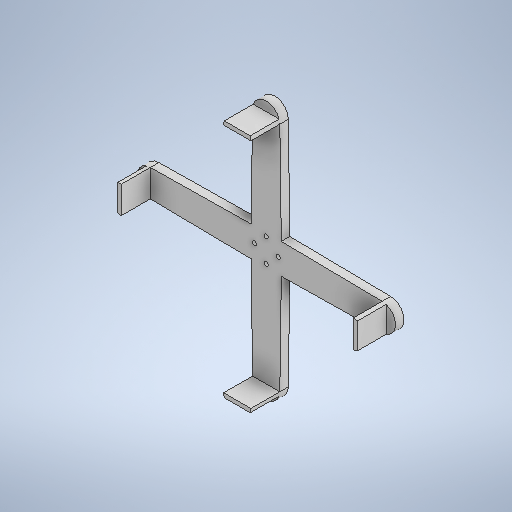
# Autodesk Inventor part: beadlock
Saved by Autodesk Inventor 2025.3 (Build 293356000, 356)
## iProperties
Created: 2026-03-16
Part Number: beadlock
Material: Generic
Document SubType Name: Modeling
Designer: ksawe
Density: 1 g/cm^3
Appearance: Default
Author: ksawe
Autodesk Inventor part; units mm, degrees
ref_plane "YZ Plane" through (0, 0, 0) normal (1, 0, 0) x (0, 1, 0)
ref_plane "XZ Plane" through (0, 0, 0) normal (0, 1, 0) x (-1, 0, 0)
ref_plane "XY Plane" through (0, 0, 0) normal (0, 0, 1) x (1, 0, 0)
sketch "Sketch1" plane through (0, 0, 0) normal (0, 0, 1) x (1, 0, 0)
  circle A0 centre (0, 0) radius 9 construction
  circle A1 centre (0, -7) radius 1.25
  circle A2 centre (7, 0) radius 1.25
  circle A3 centre (0, 7) radius 1.25
  circle A4 centre (-7, 0) radius 1.25
  circle A5 centre (0, 0) radius 60 construction
  circle A6 centre (-0.000108, -68) radius 8
  line L0 (-7.999243, -68.117634) -> (-8.999243, -0.117634)
  line L1 (8.999027, -0.132367) -> (7.999027, -68.11766)
  circle A7 centre (0, 0) radius 60 construction
  circle A8 centre (68, -0.000108) radius 8
  line L2 (0.132367, 8.999027) -> (68.11766, 7.999027)
  line L3 (68.117634, -7.999243) -> (0.117634, -8.999243)
  circle A9 centre (0, 0) radius 60 construction
  circle A10 centre (0.000108, 68) radius 8
  line L4 (-8.999027, 0.132367) -> (-7.999027, 68.11766)
  line L5 (7.999243, 68.117634) -> (8.999243, 0.117634)
  circle A11 centre (0, 0) radius 60 construction
  circle A12 centre (-68, 0.000108) radius 8
  line L6 (-0.132367, -8.999027) -> (-68.11766, -7.999027)
  line L7 (-68.117634, 7.999243) -> (-0.117634, 8.999243)
  point P0 (-8.870496, 8.870525)
  point P1 (-8.870525, -8.870496)
  point P2 (8.870496, -8.870525)
  point P3 (8.870525, 8.870496)
  dimension "d0" = 18
  dimension "d1" = 2.5
  dimension "d2" = 7
  dimension "d5" = 360
  dimension "d7" = 7
  dimension "d8" = 120
  dimension "d9" = 16
  dimension "d10" = 68
  dimension "d13" = 2.00076
  dimension "d16" = 360
  constraints: 16 end point, 12 centre point, 8 point on circle, 3 tangent, 2 coincident, 55 other
  measures "d1" diameter of A1
  measures "d2" distance of point (0, 0) A1.centre
  measures "d7" horizontal distance of A1.centre A2.centre
  measures "d8" diameter of A5
  measures "d9" diameter of A6
  measures "d10" vertical distance of L0.start L0.end
  measures "d13" distance from line of L1 A2.centre
extrude "Extrusion1" add sketch "Sketch1" along normal mid plane 5 contours A6 L0 L6 A12 L7 L4 A10 L5 L2 A8 L3 L1
extrude "Extrusion2" add sketch "Sketch1" along normal mid plane 5 contours A6 | A8 | A12 | A10
sketch "Sketch2" plane through (0, 0, 2.5) normal (0, 0, 1) x (1, 0, 0)
  arc A0 (7.999243, 68.117634) -> (-7.999027, 68.11766) centre (0.000108, 68) ccw
  line L0 (7.999243, 68.117634) -> (-7.999027, 68.11766)
  line L1 (7.603147, 70.488735) -> (-7.602931, 70.488735)
  point P0 (0, 0)
  constraints: 4 end point, 2 point on circle, 1 horizontal
extrude "Extrusion3" add sketch "Sketch2" along normal blind 17 contours L0 A0 L1
pattern_circular "Circular Pattern1" count 4 over 360 about axis through (0, 0, -10) along (0, 0, 1) of "Extrusion3"
body "Solid1"
